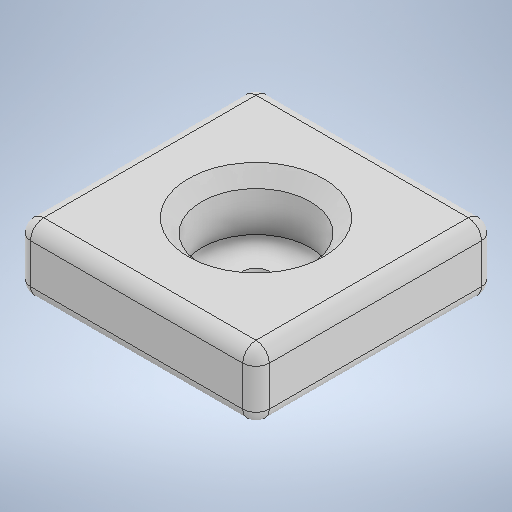
# Autodesk Inventor part: supportbalises
Saved by Autodesk Inventor 2025 (Build 290162000, 162)
## iProperties
Created: 2024-11-17
Part Number: supportbalises
Material: Generic
Document SubType Name: Modeling
Designer: Admin
Density: 1 g/cm^3
Appearance: Default
Author: Admin
## iProperties of the stored document supportbalises_3DPrint.ipt
Created: 2024-11-18
Part Number: supportbalises_3DPrint
Material: Generic
Document SubType Name: Modeling
Designer: Admin
Density: 1 g/cm^3
Appearance: Default
Author: Admin
Autodesk Inventor part; units mm, degrees
ref_plane "YZ Plane" through (0, 0, 0) normal (1, 0, 0) x (0, 1, 0)
ref_plane "XZ Plane" through (0, 0, 0) normal (0, 1, 0) x (-1, 0, 0)
ref_plane "XY Plane" through (0, 0, 0) normal (0, 0, 1) x (1, 0, 0)
sketch "Sketch1" plane through (0, 0, 0) normal (0, 1, 0) x (-1, 0, 0)
  line L0 (45, 45) -> (-45, 45)
  line L1 (-45, 45) -> (-45, -45)
  line L2 (-45, -45) -> (45, -45)
  line L3 (45, -45) -> (45, 45)
  line L4 (45, 45) -> (-45, -45)
  line L5 (45, -45) -> (-45, 45)
  point P0 (0, 0)
  point P1 (0, 0)
  dimension "d0" = 90
  dimension "d1" = 90
  constraints: 12 end point, 2 parallel, 1 coincident, 1 horizontal, 1 midpoint, 1 perpendicular
  measures "d0" distance of L2.end L0.start
  measures "d1" distance of L0.start L0.end
extrude "Extrusion1" add sketch "Sketch1" along normal blind 25
sketch "Sketch5" plane through (0, 25, 0) normal (0, 1, 0) x (1, 0, 0)
  circle A0 centre (0, 0) radius 20.5
  dimension "d27" = 41
  constraints: 1 centre point, 1 coincident
  measures "d27" diameter of A0
extrude "Extrusion3" cut sketch "Sketch5" against normal blind 20
sketch "Sketch6" plane through (0, 5, 0) normal (0, 1, 0) x (1, 0, 0)
  circle A0 centre (0, 0) radius 5
  dimension "d30" = 10
  constraints: 1 centre point, 1 coincident
  measures "d30" diameter of A0
extrude "Extrusion4" cut sketch "Sketch6" against normal blind 20
fillet "Fillet2" radius 5 8 edges at (45, 0, 0) (0, 0, -45) (-45, 0, 0) (0, 0, 45) (45, 25, 0) (0, 25, -45) (-45, 25, 0) (0, 25, 45)
chamfer "Chamfer1" distance 5 angle 45 1 edges at (-20.5, 25, 0)
fillet "Fillet3" radius 5 12 edges at (43.5355, 23.5355, 43.5355) (43.5355, 1.4645, 43.5355) (45, 12.5, 45) (43.5355, 23.5355, -43.5355) (43.5355, 1.4645, -43.5355) (45, 12.5, -45) (-43.5355, 23.5355, 43.5355) (-43.5355, 1.4645, 43.5355) (-45, 12.5, 45) (-45, 12.5, -45) (-43.5355, 1.4645, -43.5355) (-43.5355, 23.5355, -43.5355)
body "Solid1"
